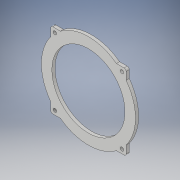
# Autodesk Inventor part: LED_Ring
Saved by Autodesk Inventor 2017 (Build 210142000, 142)
## iProperties
Part Number: LED_Ring
Material: Generisch
Document SubType Name: Modeling
Designer: Fabio
Density: 1 g/cm^3
Appearance: Vorgabe
Author: Fabio
Autodesk Inventor part; units mm, degrees
ref_plane "YZ Plane" through (0, 0, 0) normal (1, 0, 0) x (0, 1, 0)
ref_plane "XZ Plane" through (0, 0, 0) normal (0, 1, 0) x (-1, 0, 0)
ref_plane "XY Plane" through (0, 0, 0) normal (0, 0, 1) x (1, 0, 0)
sketch "Skizze1" plane through (0, 0, 0) normal (0, 1, 0) x (-1, 0, 0)
  circle A0 centre (0, 0) radius 45
  circle A1 centre (0, 0) radius 35
  dimension "d0" = 90
  dimension "d1" = 70
  constraints: 2 centre point, 2 coincident
  measures "d0" diameter of A0
  measures "d1" diameter of A1
extrude "Extrusion1" add sketch "Skizze1" along normal blind 3
sketch "Skizze6" plane through (0, 0, 0) normal (0, -1, 0) x (1, 0, 0)
  circle A0 centre (0, 0) radius 35 projected
  line L0 (-36.1127, -36.1127) -> (36.1127, -36.1127) construction
  line L1 (36.1127, -36.1127) -> (36.1127, 36.1127) construction
  line L2 (36.1127, 36.1127) -> (-36.1127, 36.1127) construction
  line L3 (-36.1127, 36.1127) -> (-36.1127, -36.1127) construction
  line L4 (-36.1127, -36.1127) -> (36.1127, 36.1127) construction
  line L5 (36.1127, -36.1127) -> (-36.1127, 36.1127) construction
  circle A1 centre (0, 0) radius 45 construction
  line L6 (-26.1127, 26.1127) -> (-36.1127, 26.1127)
  line L7 (-36.1127, 26.1127) -> (-36.1127, 36.1127)
  line L8 (-36.1127, 36.1127) -> (-26.1127, 36.1127)
  line L9 (-26.1127, 36.1127) -> (-26.1127, 26.1127)
  line L10 (-26.1127, 26.1127) -> (-36.1127, 36.1127) construction
  line L11 (-36.1127, 26.1127) -> (-26.1127, 36.1127) construction
  line L12 (-26.1127, -26.1127) -> (-26.1127, -36.1127)
  line L13 (-26.1127, -36.1127) -> (-36.1127, -36.1127)
  line L14 (-36.1127, -36.1127) -> (-36.1127, -26.1127)
  line L15 (-26.1127, -26.1127) -> (-36.1127, -36.1127) construction
  line L16 (-26.1127, -36.1127) -> (-36.1127, -26.1127) construction
  line L17 (-36.1127, -26.1127) -> (-26.1127, -26.1127)
  line L18 (26.1127, -26.1127) -> (36.1127, -26.1127)
  line L19 (36.1127, -26.1127) -> (36.1127, -36.1127)
  line L20 (36.1127, -36.1127) -> (26.1127, -36.1127)
  line L21 (26.1127, -26.1127) -> (36.1127, -36.1127) construction
  line L22 (36.1127, -26.1127) -> (26.1127, -36.1127) construction
  line L23 (26.1127, -36.1127) -> (26.1127, -26.1127)
  line L24 (26.1127, 26.1127) -> (26.1127, 36.1127)
  line L25 (26.1127, 36.1127) -> (36.1127, 36.1127)
  line L26 (36.1127, 36.1127) -> (36.1127, 26.1127)
  line L27 (26.1127, 26.1127) -> (36.1127, 36.1127) construction
  line L28 (26.1127, 36.1127) -> (36.1127, 26.1127) construction
  line L29 (36.1127, 26.1127) -> (26.1127, 26.1127)
  point P0 (-31.1127, 31.1127)
  point P1 (-31.1127, -31.1127)
  point P2 (31.1127, -31.1127)
  point P3 (31.1127, 31.1127)
  dimension "d54" = 44
  dimension "d55" = 10
  dimension "d56" = 10
  dimension "d59" = 360
  constraints: 60 end point, 10 midpoint, 4 parallel, 2 horizontal, 2 perpendicular, 1 point on line, 45 other
  measures "d54" distance of point (0, 0) point (-31.113, 31.113)
  measures "d55" distance of L6.start L6.end
  measures "d56" distance of L8.end L6.start
extrude "Extrusion4" add sketch "Skizze6" against normal blind 3 contours L6 L7 L8 L9 | L12 L13 L14 L17 | L18 L19 L20 L23 | L24 L25 L26 L29
sketch "Skizze7" plane through (0, 3, 0) normal (0, 1, 0) x (1, 0, 0)
  line L0 (-36.1127, -26.8491) -> (-36.1127, -36.1127) projected
  line L1 (-36.1127, -36.1127) -> (-26.8491, -36.1127) projected
  point P0 (0, 0)
  point P1 (-32.1127, -32.1127)
  point P2 (32.1127, -32.1127)
  point P3 (32.1127, 32.1127)
  point P4 (-32.1127, 32.1127)
  dimension "d63" = 4
  dimension "d64" = 4
  dimension "d67" = 360
  constraints: 5 other
  measures "d63" distance from line of L0 point (-32.113, -32.113)
  measures "d64" distance from line of L1 point (-32.113, -32.113)
hole "Bohrung3" at (-32.1127, 3, 32.1127) at (32.1127, 3, 32.1127) at (32.1127, 3, -32.1127) at (-32.1127, 3, -32.1127) direction (0, -1, 0) diameter 3.3 end through all
fillet "Rundung1" radius 2 4 edges at (-36.1127, 1.5, 36.1127) (-36.1127, 1.5, -36.1127) (36.1127, 1.5, 36.1127) (36.1127, 1.5, -36.1127)
